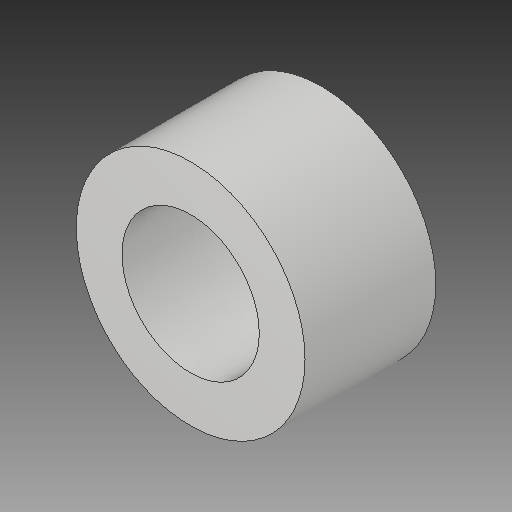
# Autodesk Inventor part: シムリング0407.4t自作
Saved by Autodesk Inventor 2020 (Build 240168000, 168)
## iProperties
Created: 2018-12-31
Part Number: シムリング0407.4t自作
Material: アルミニウム 2014-T4
Document SubType Name: Modeling
Designer: 雪村
Density: 2.8 g/cm^3
Appearance: サテン
Description: アルミ2000 4t
Mass: 0.275857 g
Surface Area: 1.90004 cm^2
Volume: 0.0985203 cm^3
Author: 雪村
Autodesk Inventor part; units mm, degrees
ref_plane "YZ Plane" through (0, 0, 0) normal (1, 0, 0) x (0, 1, 0)
ref_plane "XZ Plane" through (0, 0, 0) normal (0, 1, 0) x (-1, 0, 0)
ref_plane "XY Plane" through (0, 0, 0) normal (0, 0, 1) x (1, 0, 0)
sketch "スケッチ1" plane through (0, 0, 0) normal (0, 0, 1) x (1, 0, 0)
  circle A0 centre (0, 0) radius 2.1
  circle A1 centre (0, 0) radius 3.5
  dimension "d0" = 4.2
  dimension "d1" = 1.4
  constraints: 2 centre point, 2 coincident
  measures "d0" diameter of A0
  measures "d1" radial gap between concentric circles of A1 A0
extrude "押し出し1" add sketch "スケッチ1" along normal blind 4
